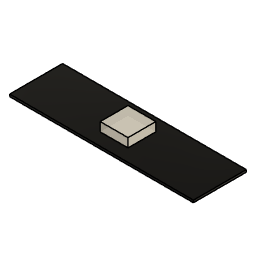
led_solderRig v2 (Autodesk Fusion 360 archive; units mm, degrees)
design "led"
Autodesk Fusion 360 part; units mm, degrees
sketch "Sketch1" plane through (0, 0, 0) normal (0, 0, 1) x (1, 0, 0)
  line L0 (16.5, -4.75) -> (-16.5, -4.75)
  line L1 (-16.5, -4.75) -> (-16.5, 4.75)
  line L2 (-16.5, 4.75) -> (16.5, 4.75)
  line L3 (16.5, 4.75) -> (16.5, -4.75)
  line L4 (16.5, -4.75) -> (-16.5, 4.75) construction
  line L5 (-16.5, -4.75) -> (16.5, 4.75) construction
  line L6 (2.5, -2.5) -> (-2.5, -2.5)
  line L7 (-2.5, -2.5) -> (-2.5, 2.5)
  line L8 (-2.5, 2.5) -> (2.5, 2.5)
  line L9 (2.5, 2.5) -> (2.5, -2.5)
  line L10 (2.5, -2.5) -> (-2.5, 2.5) construction
  line L11 (-2.5, -2.5) -> (2.5, 2.5) construction
  dimension "d1" = 14
  dimension "d2" = 14
  dimension "d3" = 5
  dimension "d4" = 5
  dimension "d5" = 9.5
  dimension "d6" = 33
  constraint horizontal L0
  constraint perpendicular L0 L1
  constraint parallel L0 L2
  constraint parallel L1 L3
  constraint coincident L4 origin
  constraint coincident L5 origin
  constraint horizontal L6
  constraint perpendicular L6 L7
  constraint parallel L6 L8
  constraint parallel L7 L9
  constraint coincident L10 origin
  constraint coincident L11 origin
  measures "d1" distance of L3 L9
  measures "d2" distance of L1 L7
  measures "d3" distance of L7.end L8.end
  measures "d4" distance of L6.start L8.end
  measures "d5" distance of L0.start L2.end
  measures "d6" distance of L0.start L0.end
extrude "Extrude1" add sketch "Sketch1" against normal blind 0.4 contours L0 L1 L2 L3 | L6 L7 L8 L9
extrude "Extrude2" add sketch "Sketch1" along normal blind 1.6 contours L6 L7 L8 L9
